Autodesk Fusion 360 part; units mm, degrees
note: some values were not read from the file. Set by a fixed rule: which sketch regions a step uses.
(part 2 of 2)
sketch "Sketch21" plane through (0, 0, -10) normal (0, 0, -1) x (1, 0, 0)
  spline S0 degree 3 poles (20.862, 26.2779) (22.0749, 27.628) (22.1899, 27.6698) (22.8451, 26.9999) knots 0 0 0 0 1 1 1 1
  spline S1 degree 3 poles (22.8451, 26.9999) (23.28, 26.5551) (23.2541, 26.3604) (22.6927, 25.8492) knots 0 0 0 0 1 1 1 1
  spline S2 degree 3 poles (22.6927, 25.8492) (21.2501, 24.5364) (20.8273, 24.3583) (20.2979, 24.842) knots 0 0 0 0 1 1 1 1
  spline S3 degree 3 poles (20.2979, 24.842) (19.869, 25.2336) (19.8267, 25.1253) (20.862, 26.2779) knots 0 0 0 0 1 1 1 1
  spline S4 degree 3 poles (14.6678, 20.2808) (15.0237, 20.7097) (15.5235, 21.3317) (17.1491, 23.3698) knots 0 0 0 0 1 1 1 1
  spline S5 degree 3 poles (17.1491, 23.3698) (17.5034, 23.8143) (17.8222, 24.1162) (17.9402, 24.1191) knots 0 0 0 0 1 1 1 1
  spline S6 degree 3 poles (17.9402, 24.1191) (18.2344, 24.1265) (19.9603, 22.9367) (20.9237, 22.0623) knots 0 0 0 0 1 1 1 1
  spline S7 degree 3 poles (20.9237, 22.0623) (20.9678, 22.0223) (20.8255, 21.7837) (20.6075, 21.5323) knots 0 0 0 0 1 1 1 1
  spline S8 degree 3 poles (20.6075, 21.5323) (20.3895, 21.2809) (19.9532, 20.7497) (19.6383, 20.3517) knots 0 0 0 0 1 1 1 1
  spline S9 degree 3 poles (19.6383, 20.3517) (18.9242, 19.4495) (17.0861, 17.5096) (16.9451, 17.5096) knots 0 0 0 0 1 1 1 1
  spline S10 degree 3 poles (16.9451, 17.5096) (16.8874, 17.5096) (16.566, 17.7633) (16.231, 18.0737) knots 0 0 0 0 1 1 1 1
  spline S11 degree 3 poles (16.231, 18.0737) (15.8958, 18.3838) (15.32, 18.8531) (14.9509, 19.1161) knots 0 0 0 0 1 1 1 1
  spline S12 degree 3 poles (14.9509, 19.1161) (14.1651, 19.677) (14.1654, 19.6755) (14.6678, 20.2808) knots 0 0 0 0 1 1 1 1
  spline S13 degree 3 poles (29.4215, 8.4259) (29.9899, 8.5418) (30.8969, 8.731) (31.4369, 8.8463) knots 0 0 0 0 1 1 1 1
  spline S14 degree 3 poles (31.4369, 8.8463) (31.9769, 8.9617) (32.628, 9.0921) (32.8839, 9.1363) knots 0 0 0 0 1 1 1 1
  spline S15 degree 3 poles (32.8839, 9.1363) (33.4104, 9.2273) (34.532, 9.444) (36.3462, 9.8054) knots 0 0 0 0 1 1 1 1
  spline S16 degree 3 poles (36.3462, 9.8054) (38.5867, 10.2521) (38.883, 10.3047) (38.9201, 10.2637) knots 0 0 0 0 1 1 1 1
  spline S17 degree 3 poles (38.9201, 10.2637) (39.3336, 9.807) (39.7083, 7.5488) (39.3982, 7.3826) knots 0 0 0 0 1 1 1 1
  spline S18 degree 3 poles (39.3982, 7.3826) (39.0804, 7.2128) (37.4413, 6.8204) (35.0543, 6.3428) knots 0 0 0 0 1 1 1 1
  spline S19 degree 3 poles (35.0543, 6.3428) (33.9459, 6.1211) (32.1086, 5.7496) (30.9717, 5.5173) knots 0 0 0 0 1 1 1 1
  spline S20 degree 3 poles (30.9717, 5.5173) (26.6447, 4.6334) (23.86, 4.1852) (23.7544, 4.3558) knots 0 0 0 0 1 1 1 1
  spline S21 degree 3 poles (23.7544, 4.3558) (23.6788, 4.4786) (23.2549, 6.4365) (23.2356, 6.7529) knots 0 0 0 0 1 1 1 1
  spline S22 degree 3 poles (23.2356, 6.7529) (23.2218, 6.9792) (23.2901, 7.0215) (23.9439, 7.1921) knots 0 0 0 0 1 1 1 1
  spline S23 degree 3 poles (23.9439, 7.1921) (25.0588, 7.4832) (27.5544, 8.0452) (29.4215, 8.4259) knots 0 0 0 0 1 1 1 1
  spline S24 degree 3 poles (31.5403, -12.6172) (31.5403, -12.6934) (31.5618, -12.8178) (31.5882, -12.8934) knots 0 0 0 0 1 1 1 1
  spline S25 degree 3 poles (31.5882, -12.8934) (31.6147, -12.9691) (31.5742, -13.1728) (31.4985, -13.3461) knots 0 0 0 0 1 1 1 1
  spline S26 degree 3 poles (31.4985, -13.3461) (31.0239, -14.4338) (29.3639, -14.115) (29.3734, -12.9379) knots 0 0 0 0 1 1 1 1
  spline S27 degree 3 poles (29.3734, -12.9379) (29.3813, -11.9494) (30.5288, -11.4671) (31.2223, -12.1605) knots 0 0 0 0 1 1 1 1
  spline S28 degree 3 poles (31.2223, -12.1605) (31.3972, -12.3354) (31.5403, -12.541) (31.5403, -12.6172) knots 0 0 0 0 1 1 1 1
  line L0 (15.4452, -28.439) -> (15.3796, -27.5151)
  spline S29 degree 3 poles (15.3796, -27.5151) (15.2729, -26.0133) (15.9352, -25.8345) (17.2002, -27.0232) knots 0 0 0 0 1 1 1 1
  spline S30 degree 3 poles (17.2002, -27.0232) (17.6648, -27.4601) (17.6664, -27.5019) (17.2568, -28.461) knots 0 0 0 0 1 1 1 1
  spline S31 degree 3 poles (17.2568, -28.461) (17.0798, -28.8756) (16.8843, -29.201) (16.8221, -29.1844) knots 0 0 0 0 1 1 1 1
  spline S32 degree 3 poles (16.8221, -29.1844) (16.7599, -29.1677) (16.4247, -28.9933) (16.077, -28.7965) knots 0 0 0 0 1 1 1 1
  line L1 (16.077, -28.7965) -> (15.4452, -28.439)
  line L2 (2.2258, -22.5912) -> (3.0868, -22.5912)
  line L3 (3.0868, -22.5912) -> (3.2683, -23.6506)
  spline S33 degree 3 poles (3.2683, -23.6506) (3.3683, -24.2332) (3.608, -25.3561) (3.8009, -26.1456) knots 0 0 0 0 1 1 1 1
  spline S34 degree 3 poles (3.8009, -26.1456) (4.2713, -28.0697) (4.2668, -28.1578) (3.6768, -28.6525) knots 0 0 0 0 1 1 1 1
  spline S35 degree 3 poles (3.6768, -28.6525) (3.0362, -29.1894) (2.588, -29.3391) (1.8387, -29.2659) knots 0 0 0 0 1 1 1 1
  spline S36 degree 3 poles (1.8387, -29.2659) (0.3557, -29.1206) (-0.1128, -28.1046) (0.4711, -26.2993) knots 0 0 0 0 1 1 1 1
  spline S37 degree 3 poles (0.4711, -26.2993) (0.6719, -25.6781) (1.0444, -24.1485) (1.3172, -22.8238) knots 0 0 0 0 1 1 1 1
  spline S38 degree 3 poles (1.3172, -22.8238) (1.3622, -22.6052) (1.4165, -22.5912) (2.2258, -22.5912) knots 0 0 0 0 1 1 1 1
  spline S39 degree 3 poles (-30.4455, 10.3042) (-30.1303, 10.7241) (-28.6807, 10.95) (-28.36, 10.6293) knots 0 0 0 0 1 1 1 1
  spline S40 degree 3 poles (-28.36, 10.6293) (-28.1904, 10.4597) (-28.0986, -8.8151) (-28.2666, -8.9832) knots 0 0 0 0 1 1 1 1
  spline S41 degree 3 poles (-28.2666, -8.9832) (-28.3537, -9.0702) (-29.8806, -9.0739) (-30.1049, -8.9879) knots 0 0 0 0 1 1 1 1
  spline S42 degree 3 poles (-30.1049, -8.9879) (-30.5796, -8.8056) (-30.5748, -8.9072) (-30.5748, 0.8967) knots 0 0 0 0 1 1 1 1
  spline S43 degree 3 poles (-30.5748, 0.8967) (-30.5748, 8.1243) (-30.5468, 10.1695) (-30.4455, 10.3042) knots 0 0 0 0 1 1 1 1
  spline S44 degree 3 poles (-13.179, 9.603) (-13.0383, 9.2054) (-12.7991, 8.4378) (-12.6472, 7.8978) knots 0 0 0 0 1 1 1 1
  spline S45 degree 3 poles (-12.6472, 7.8978) (-12.4951, 7.3578) (-12.349, 6.8389) (-12.3223, 6.7447) knots 0 0 0 0 1 1 1 1
  spline S46 degree 3 poles (-12.3223, 6.7447) (-12.104, 5.9769) (-17.0523, 3.5076) (-19.3094, 3.2581) knots 0 0 0 0 1 1 1 1
  line L4 (-19.3094, 3.2581) -> (-19.8777, 3.1953)
  line L5 (-19.8777, 3.1953) -> (-19.8777, -1.4539)
  line L6 (-19.8777, -1.4539) -> (-19.1025, -1.5682)
  spline S47 degree 3 poles (-19.1025, -1.5682) (-16.6231, -1.9341) (-13.6717, -3.4131) (-12.0702, -5.0925) knots 0 0 0 0 1 1 1 1
  spline S48 degree 3 poles (-12.0702, -5.0925) (-10.9073, -6.3114) (-9.4825, -8.0603) (-9.1812, -8.6387) knots 0 0 0 0 1 1 1 1
  spline S49 degree 3 poles (-9.1812, -8.6387) (-9.1071, -8.7808) (-9.0134, -8.9202) (-8.9729, -8.9488) knots 0 0 0 0 1 1 1 1
  spline S50 degree 3 poles (-8.9729, -8.9488) (-8.4647, -9.3062) (-8.1371, -13.3914) (-8.32, -17.0871) knots 0 0 0 0 1 1 1 1
  line L7 (-8.32, -17.0871) -> (-8.3623, -17.939)
  line L8 (-8.3623, -17.939) -> (-8.9568, -17.639)
  spline S51 degree 3 poles (-8.9568, -17.639) (-10.9986, -16.6085) (-12.788, -15.0109) (-14.5231, -12.6693) knots 0 0 0 0 1 1 1 1
  spline S52 degree 3 poles (-14.5231, -12.6693) (-16.5808, -9.8931) (-18.1228, -8.994) (-21.0377, -8.872) knots 0 0 0 0 1 1 1 1
  line L9 (-21.0377, -8.872) -> (-22.4098, -8.8144)
  line L10 (-22.4098, -8.8144) -> (-22.4098, 0.7612)
  spline S53 degree 3 poles (-22.4098, 0.7612) (-22.4098, 8.0711) (-22.3804, 10.3664) (-22.286, 10.4611) knots 0 0 0 0 1 1 1 1
  spline S54 degree 3 poles (-22.286, 10.4611) (-22.2063, 10.5404) (-21.8005, 10.5849) (-21.1557, 10.5849) knots 0 0 0 0 1 1 1 1
  spline S55 degree 3 poles (-21.1557, 10.5849) (-18.3574, 10.5849) (-15.9831, 11.8954) (-14.8821, 14.0472) knots 0 0 0 0 1 1 1 1
  spline S56 degree 3 poles (-14.8821, 14.0472) (-14.6784, 14.4457) (-14.5633, 14.5896) (-14.5602, 14.4494) knots 0 0 0 0 1 1 1 1
  spline S57 degree 3 poles (-14.5602, 14.4494) (-14.5541, 14.1856) (-13.5365, 10.6153) (-13.179, 9.603) knots 0 0 0 0 1 1 1 1
  spline S58 degree 3 poles (-5.6836, 12.591) (-5.958, 12.4497) (-5.9604, 12.4518) (-6.3298, 13.1654) knots 0 0 0 0 1 1 1 1
  spline S59 degree 3 poles (-6.3298, 13.1654) (-6.7885, 14.052) (-6.788, 14.0732) (-6.3128, 14.27) knots 0 0 0 0 1 1 1 1
  spline S60 degree 3 poles (-6.3128, 14.27) (-6.0996, 14.3584) (-5.7366, 14.5155) (-5.5061, 14.6198) knots 0 0 0 0 1 1 1 1
  spline S61 degree 3 poles (-5.5061, 14.6198) (-2.2832, 16.0763) (2.9227, 16.2012) (5.8226, 14.8915) knots 0 0 0 0 1 1 1 1
  spline S62 degree 3 poles (5.8226, 14.8915) (6.012, 14.8058) (6.4843, 14.5925) (6.8719, 14.4174) knots 0 0 0 0 1 1 1 1
  spline S63 degree 3 poles (6.8719, 14.4174) (7.2598, 14.2422) (7.5961, 14.0991) (7.6199, 14.0991) knots 0 0 0 0 1 1 1 1
  spline S64 degree 3 poles (7.6199, 14.0991) (8.0964, 14.0991) (10.6404, 12.052) (11.7939, 10.7399) knots 0 0 0 0 1 1 1 1
  spline S65 degree 3 poles (11.7939, 10.7399) (14.2884, 7.9039) (15.8315, 2.9054) (15.3518, -0.7837) knots 0 0 0 0 1 1 1 1
  spline S66 degree 3 poles (15.3518, -0.7837) (15.3261, -0.9827) (15.1899, -1.7124) (15.0494, -2.4054) knots 0 0 0 0 1 1 1 1
  spline S67 degree 3 poles (15.0494, -2.4054) (14.7007, -4.1254) (14.3112, -5.1134) (13.101, -7.348) knots 0 0 0 0 1 1 1 1
  spline S68 degree 3 poles (13.101, -7.348) (11.2545, -10.758) (6.6772, -13.6369) (2.5756, -13.9684) knots 0 0 0 0 1 1 1 1
  line L11 (2.5756, -13.9684) -> (1.6712, -14.0415)
  line L12 (1.6712, -14.0415) -> (1.6712, -13.6139)
  spline S69 degree 3 poles (1.6712, -13.6139) (1.6712, -13.3416) (1.7183, -13.1855) (1.8006, -13.1842) knots 0 0 0 0 1 1 1 1
  spline S70 degree 3 poles (1.8006, -13.1842) (8.8176, -13.0747) (14.7896, -6.5384) (14.4522, 0.663) knots 0 0 0 0 1 1 1 1
  spline S71 degree 3 poles (14.4522, 0.663) (13.9887, 10.5569) (3.0063, 17.0624) (-5.6836, 12.591) knots 0 0 0 0 1 1 1 1
  spline S72 degree 3 poles (-26.4402, 11.3101) (-26.1328, 12.3822) (-24.7717, 12.4981) (-24.26, 11.4953) knots 0 0 0 0 1 1 1 1
  spline S73 degree 3 poles (-24.26, 11.4953) (-24.0473, 11.0778) (-23.9563, -9.3226) (-24.1651, -9.8394) knots 0 0 0 0 1 1 1 1
  spline S74 degree 3 poles (-24.1651, -9.8394) (-24.5095, -10.6921) (-26.1336, -10.7379) (-26.4508, -9.9039) knots 0 0 0 0 1 1 1 1
  spline S75 degree 3 poles (-26.4508, -9.9039) (-26.5804, -9.5629) (-26.5704, 10.8564) (-26.4402, 11.3101) knots 0 0 0 0 1 1 1 1
  spline S76 degree 3 poles (4.9979, -22.0247) (5.0264, -21.9996) (7.2714, -21.4088) (7.8252, -21.2807) knots 0 0 0 0 1 1 1 1
  spline S77 degree 3 poles (7.8252, -21.2807) (8.0054, -21.2389) (8.0636, -21.3201) (8.2207, -21.834) knots 0 0 0 0 1 1 1 1
  spline S78 degree 3 poles (8.2207, -21.834) (9.0079, -24.4055) (11.1888, -31.0486) (12.3091, -34.2876) knots 0 0 0 0 1 1 1 1
  spline S79 degree 3 poles (12.3091, -34.2876) (12.5975, -35.1213) (12.8335, -35.8222) (12.8335, -35.8452) knots 0 0 0 0 1 1 1 1
  spline S80 degree 3 poles (12.8335, -35.8452) (12.8335, -35.8683) (12.6126, -35.9857) (12.3424, -36.1067) knots 0 0 0 0 1 1 1 1
  spline S81 degree 3 poles (12.3424, -36.1067) (10.7356, -36.8261) (10.1498, -37.0345) (10.0562, -36.9205) knots 0 0 0 0 1 1 1 1
  spline S82 degree 3 poles (10.0562, -36.9205) (10.003, -36.8554) (9.795, -36.3138) (9.5942, -35.7172) knots 0 0 0 0 1 1 1 1
  spline S83 degree 3 poles (9.5942, -35.7172) (9.3936, -35.1203) (8.9177, -33.7482) (8.5369, -32.6681) knots 0 0 0 0 1 1 1 1
  spline S84 degree 3 poles (8.5369, -32.6681) (7.8972, -30.8536) (6.5777, -27.0262) (5.8292, -24.8134) knots 0 0 0 0 1 1 1 1
  spline S85 degree 3 poles (5.8292, -24.8134) (5.4048, -23.5593) (4.9579, -22.0599) (4.9979, -22.0247) knots 0 0 0 0 1 1 1 1
  spline S86 degree 3 poles (21.0387, -22.9492) (21.6407, -22.859) (21.9426, -23.028) (22.962, -24.026) knots 0 0 0 0 1 1 1 1
  spline S87 degree 3 poles (22.962, -24.026) (23.964, -25.0066) (23.9616, -24.9203) (22.9998, -25.4686) knots 0 0 0 0 1 1 1 1
  spline S88 degree 3 poles (22.9998, -25.4686) (22.0664, -26.0006) (22.2111, -26.0856) (21.2099, -24.4197) knots 0 0 0 0 1 1 1 1
  spline S89 degree 3 poles (21.2099, -24.4197) (20.4003, -23.0722) (20.3971, -23.0455) (21.0387, -22.9492) knots 0 0 0 0 1 1 1 1
  line L13 (22.7035, -7.4025) -> (23.4271, -7.7206)
  spline S90 degree 3 poles (23.4271, -7.7206) (23.8251, -7.8957) (24.3831, -8.1471) (24.6672, -8.2794) knots 0 0 0 0 1 1 1 1
  spline S91 degree 3 poles (24.6672, -8.2794) (24.9517, -8.4114) (25.6025, -8.6911) (26.1142, -8.9003) knots 0 0 0 0 1 1 1 1
  spline S92 degree 3 poles (26.1142, -8.9003) (27.3837, -9.42) (28.1306, -9.7766) (28.1246, -9.8605) knots 0 0 0 0 1 1 1 1
  spline S93 degree 3 poles (28.1246, -9.8605) (28.1216, -9.8991) (27.9454, -10.3026) (27.7324, -10.7575) knots 0 0 0 0 1 1 1 1
  spline S94 degree 3 poles (27.7324, -10.7575) (27.5197, -11.212) (27.189, -11.9214) (26.9974, -12.3336) knots 0 0 0 0 1 1 1 1
  spline S95 degree 3 poles (26.9974, -12.3336) (26.5762, -13.2395) (26.5648, -13.2398) (24.9194, -12.3643) knots 0 0 0 0 1 1 1 1
  spline S96 degree 3 poles (24.9194, -12.3643) (24.8305, -12.3172) (24.0166, -11.9026) (23.1107, -11.443) knots 0 0 0 0 1 1 1 1
  spline S97 degree 3 poles (23.1107, -11.443) (22.2045, -10.9834) (21.4028, -10.5672) (21.3285, -10.5177) knots 0 0 0 0 1 1 1 1
  spline S98 degree 3 poles (21.3285, -10.5177) (21.2247, -10.4487) (21.3674, -10.0799) (21.9486, -8.9154) knots 0 0 0 0 1 1 1 1
  line L14 (21.9486, -8.9154) -> (22.7035, -7.4025)
  spline S99 degree 3 poles (33.5832, 1.5933) (34.3782, 1.5933) (34.8585, 0.8376) (34.5679, 0.0431) knots 0 0 0 0 1 1 1 1
  spline S100 degree 3 poles (34.5679, 0.0431) (34.242, -0.8485) (32.9074, -0.7922) (32.6291, 0.1249) knots 0 0 0 0 1 1 1 1
  spline S101 degree 3 poles (32.6291, 0.1249) (32.3986, 0.8837) (32.8598, 1.5933) (33.5832, 1.5933) knots 0 0 0 0 1 1 1 1
  spline S102 degree 3 poles (18.3254, 16.1044) (18.993, 16.6134) (22.1595, 18.9637) (22.4453, 19.1624) knots 0 0 0 0 1 1 1 1
  spline S103 degree 3 poles (22.4453, 19.1624) (22.6442, 19.3008) (22.8535, 19.4699) (22.9104, 19.5381) knots 0 0 0 0 1 1 1 1
  spline S104 degree 3 poles (22.9104, 19.5381) (22.9673, 19.6064) (23.1768, 19.771) (23.3763, 19.9038) knots 0 0 0 0 1 1 1 1
  spline S105 degree 3 poles (23.3763, 19.9038) (23.5756, 20.0366) (24.3116, 20.5637) (25.0117, 21.0754) knots 0 0 0 0 1 1 1 1
  spline S106 degree 3 poles (25.0117, 21.0754) (25.7116, 21.5868) (26.3857, 22.0739) (26.5093, 22.1575) knots 0 0 0 0 1 1 1 1
  spline S107 degree 3 poles (26.5093, 22.1575) (26.7807, 22.3406) (28.4087, 23.5318) (29.4562, 24.3136) knots 0 0 0 0 1 1 1 1
  line L15 (29.4562, 24.3136) -> (30.2142, 24.8793)
  line L16 (30.2142, 24.8793) -> (30.7418, 24.7573)
  spline S108 degree 3 poles (30.7418, 24.7573) (32.1319, 24.4366) (32.8736, 22.9925) (32.0311, 22.2477) knots 0 0 0 0 1 1 1 1
  spline S109 degree 3 poles (32.0311, 22.2477) (31.8464, 22.0845) (30.7979, 21.2886) (29.7007, 20.4795) knots 0 0 0 0 1 1 1 1
  spline S110 degree 3 poles (29.7007, 20.4795) (28.6037, 19.6704) (27.5517, 18.892) (27.3631, 18.7499) knots 0 0 0 0 1 1 1 1
  spline S111 degree 3 poles (27.3631, 18.7499) (27.1744, 18.6079) (26.5143, 18.1231) (25.896, 17.6728) knots 0 0 0 0 1 1 1 1
  spline S112 degree 3 poles (25.896, 17.6728) (25.2779, 17.2225) (24.7088, 16.7907) (24.6313, 16.7132) knots 0 0 0 0 1 1 1 1
  spline S113 degree 3 poles (24.6313, 16.7132) (24.5537, 16.6357) (24.2278, 16.3896) (23.9071, 16.1665) knots 0 0 0 0 1 1 1 1
  spline S114 degree 3 poles (23.9071, 16.1665) (23.5862, 15.9432) (22.626, 15.2469) (21.7735, 14.619) knots 0 0 0 0 1 1 1 1
  line L17 (21.7735, 14.619) -> (20.223, 13.4776)
  line L18 (20.223, 13.4776) -> (19.9648, 13.8014)
  spline S115 degree 3 poles (19.9648, 13.8014) (19.8227, 13.9798) (19.3623, 14.5454) (18.9417, 15.0582) knots 0 0 0 0 1 1 1 1
  spline S116 degree 3 poles (18.9417, 15.0582) (18.3106, 15.8279) (18.2027, 16.011) (18.3254, 16.1044) knots 0 0 0 0 1 1 1 1
  spline S117 degree 3 poles (5.041, 26.8875) (5.458, 28.5226) (5.9133, 30.2789) (6.053, 30.7906) knots 0 0 0 0 1 1 1 1
  spline S118 degree 3 poles (6.053, 30.7906) (6.1927, 31.302) (6.5406, 32.581) (6.8261, 33.6328) knots 0 0 0 0 1 1 1 1
  spline S119 degree 3 poles (6.8261, 33.6328) (8.0051, 37.9764) (8.1922, 38.4902) (8.5946, 38.4902) knots 0 0 0 0 1 1 1 1
  spline S120 degree 3 poles (8.5946, 38.4902) (9.0468, 38.4902) (10.9827, 37.6023) (10.9608, 37.4052) knots 0 0 0 0 1 1 1 1
  spline S121 degree 3 poles (10.9608, 37.4052) (10.9544, 37.3483) (10.5615, 35.7902) (10.0874, 33.9428) knots 0 0 0 0 1 1 1 1
  spline S122 degree 3 poles (10.0874, 33.9428) (9.6132, 32.0953) (9.1568, 30.2815) (9.0735, 29.9119) knots 0 0 0 0 1 1 1 1
  spline S123 degree 3 poles (9.0735, 29.9119) (8.6557, 28.0617) (7.3971, 23.2301) (7.3024, 23.1121) knots 0 0 0 0 1 1 1 1
  spline S124 degree 3 poles (7.3024, 23.1121) (7.2891, 23.0957) (7.0978, 23.1521) (6.8777, 23.2381) knots 0 0 0 0 1 1 1 1
  spline S125 degree 3 poles (6.8777, 23.2381) (6.5322, 23.3725) (5.4476, 23.6606) (4.5534, 23.8556) knots 0 0 0 0 1 1 1 1
  line L19 (4.5534, 23.8556) -> (4.2835, 23.9143)
  line L20 (4.2835, 23.9143) -> (5.041, 26.8875)
  line L21 (-0.2801, 34.5887) -> (-0.2925, 35.2864)
  line L22 (-0.2925, 35.2864) -> (0.1986, 35.307)
  spline S126 degree 3 poles (0.1986, 35.307) (1.0609, 35.3433) (1.2971, 35.3073) (1.435, 35.1186) knots 0 0 0 0 1 1 1 1
  spline S127 degree 3 poles (1.435, 35.1186) (1.6403, 34.8379) (1.7829, 34.2323) (1.6744, 34.1016) knots 0 0 0 0 1 1 1 1
  spline S128 degree 3 poles (1.6744, 34.1016) (1.6228, 34.0394) (1.5847, 33.8365) (1.59, 33.6507) knots 0 0 0 0 1 1 1 1
  spline S129 degree 3 poles (1.59, 33.6507) (1.6011, 33.2592) (1.5125, 33.1467) (1.1545, 33.0988) knots 0 0 0 0 1 1 1 1
  spline S130 degree 3 poles (1.1545, 33.0988) (0.8693, 33.0607) (0.8479, 32.8271) (0.9987, 31.3946) knots 0 0 0 0 1 1 1 1
  line L23 (0.9987, 31.3946) -> (1.0656, 30.7583)
  line L24 (1.0656, 30.7583) -> (1.7043, 30.6459)
  spline S131 degree 3 poles (1.7043, 30.6459) (2.6597, 30.4779) (3.0116, 30.1262) (2.8526, 29.4986) knots 0 0 0 0 1 1 1 1
  spline S132 degree 3 poles (2.8526, 29.4986) (2.8312, 29.4132) (2.7685, 28.5993) (2.7137, 27.6899) knots 0 0 0 0 1 1 1 1
  spline S133 degree 3 poles (2.7137, 27.6899) (2.6126, 26.0162) (2.4377, 24.6144) (2.2949, 24.3311) knots 0 0 0 0 1 1 1 1
  spline S134 degree 3 poles (2.2949, 24.3311) (2.2237, 24.1898) (-0.4422, 24.149) (-0.5901, 24.2869) knots 0 0 0 0 1 1 1 1
  spline S135 degree 3 poles (-0.5901, 24.2869) (-0.6722, 24.3633) (-1.1159, 28.5496) (-1.1175, 29.2616) knots 0 0 0 0 1 1 1 1
  line L25 (-1.1175, 29.2616) -> (-1.1193, 30.0066)
  line L26 (-1.1193, 30.0066) -> (-0.6648, 30.2728)
  spline S136 degree 3 poles (-0.6648, 30.2728) (-0.415, 30.4194) (-0.0078, 30.5736) (0.2396, 30.6154) knots 0 0 0 0 1 1 1 1
  spline S137 degree 3 poles (0.2396, 30.6154) (0.7621, 30.7043) (0.823, 30.9493) (0.6671, 32.3408) knots 0 0 0 0 1 1 1 1
  spline S138 degree 3 poles (0.6671, 32.3408) (0.5875, 33.052) (0.5798, 33.0663) (0.2242, 33.1808) knots 0 0 0 0 1 1 1 1
  spline S139 degree 3 poles (0.2242, 33.1808) (-0.1941, 33.3158) (-0.2613, 33.5034) (-0.2801, 34.5887) knots 0 0 0 0 1 1 1 1
  spline S140 degree 3 poles (9.6302, 23.2471) (9.9683, 23.9704) (10.2721, 24.7504) (10.8367, 26.3464) knots 0 0 0 0 1 1 1 1
  spline S141 degree 3 poles (10.8367, 26.3464) (11.301, 27.6582) (11.1788, 27.5934) (12.3189, 27.1346) knots 0 0 0 0 1 1 1 1
  spline S142 degree 3 poles (12.3189, 27.1346) (14.8602, 26.112) (14.988, 25.9866) (14.5416, 24.951) knots 0 0 0 0 1 1 1 1
  spline S143 degree 3 poles (14.5416, 24.951) (13.8572, 23.3632) (12.8158, 21.2952) (12.4723, 20.8415) knots 0 0 0 0 1 1 1 1
  spline S144 degree 3 poles (12.4723, 20.8415) (12.4308, 20.7864) (11.7246, 21.1254) (10.824, 21.6326) knots 0 0 0 0 1 1 1 1
  spline S145 degree 3 poles (10.824, 21.6326) (10.3154, 21.9186) (9.7691, 22.1816) (9.6095, 22.2165) knots 0 0 0 0 1 1 1 1
  spline S146 degree 3 poles (9.6095, 22.2165) (9.2436, 22.2969) (9.2463, 22.4261) (9.6302, 23.2471) knots 0 0 0 0 1 1 1 1
  spline S147 degree 3 poles (22.3442, 9.3869) (22.3423, 9.4578) (21.4819, 11.2911) (21.2385, 11.7422) knots 0 0 0 0 1 1 1 1
  spline S148 degree 3 poles (21.2385, 11.7422) (21.1896, 11.8332) (26.3783, 14.4092) (26.6101, 14.4092) knots 0 0 0 0 1 1 1 1
  spline S149 degree 3 poles (26.6101, 14.4092) (26.8159, 14.4092) (27.0001, 14.1345) (27.3033, 13.3755) knots 0 0 0 0 1 1 1 1
  spline S150 degree 3 poles (27.3033, 13.3755) (27.4282, 13.063) (27.6885, 12.4428) (27.8817, 11.9975) knots 0 0 0 0 1 1 1 1
  spline S151 degree 3 poles (27.8817, 11.9975) (28.2976, 11.0384) (28.2997, 11.0212) (28.0005, 10.8987) knots 0 0 0 0 1 1 1 1
  spline S152 degree 3 poles (28.0005, 10.8987) (27.8727, 10.8463) (27.326, 10.6336) (26.786, 10.4259) knots 0 0 0 0 1 1 1 1
  spline S153 degree 3 poles (26.786, 10.4259) (26.246, 10.2184) (25.7576, 10.0137) (25.701, 9.9708) knots 0 0 0 0 1 1 1 1
  spline S154 degree 3 poles (25.701, 9.9708) (25.601, 9.8959) (24.2693, 9.3591) (23.2348, 8.9768) knots 0 0 0 0 1 1 1 1
  line L27 (23.2348, 8.9768) -> (22.7323, 8.791)
  line L28 (22.7323, 8.791) -> (22.5395, 9.0421)
  spline S155 degree 3 poles (22.5395, 9.0421) (22.4334, 9.1802) (22.3455, 9.3353) (22.3442, 9.3869) knots 0 0 0 0 1 1 1 1
  spline S156 degree 3 poles (23.1811, -5.6857) (23.1184, -5.6161) (23.7126, -3.1007) (23.8452, -2.875) knots 0 0 0 0 1 1 1 1
  spline S157 degree 3 poles (23.8452, -2.875) (23.8542, -2.8596) (24.4847, -2.9898) (25.2462, -3.1642) knots 0 0 0 0 1 1 1 1
  spline S158 degree 3 poles (25.2462, -3.1642) (26.0079, -3.3385) (26.9686, -3.5481) (27.3813, -3.6296) knots 0 0 0 0 1 1 1 1
  spline S159 degree 3 poles (27.3813, -3.6296) (27.7941, -3.7113) (28.5847, -3.8902) (29.1384, -4.0272) knots 0 0 0 0 1 1 1 1
  spline S160 degree 3 poles (29.1384, -4.0272) (29.6919, -4.1643) (30.7961, -4.4257) (31.5919, -4.6083) knots 0 0 0 0 1 1 1 1
  spline S161 degree 3 poles (31.5919, -4.6083) (36.0499, -5.6306) (39.4024, -6.5403) (39.3844, -6.7226) knots 0 0 0 0 1 1 1 1
  spline S162 degree 3 poles (39.3844, -6.7226) (39.3786, -6.7816) (39.3085, -7.3184) (39.2286, -7.915) knots 0 0 0 0 1 1 1 1
  spline S163 degree 3 poles (39.2286, -7.915) (39.1487, -8.5119) (39.0619, -9.0586) (39.0357, -9.1295) knots 0 0 0 0 1 1 1 1
  spline S164 degree 3 poles (39.0357, -9.1295) (38.978, -9.2864) (37.93, -9.3046) (37.2963, -9.1596) knots 0 0 0 0 1 1 1 1
  spline S165 degree 3 poles (37.2963, -9.1596) (37.0579, -9.1051) (36.3745, -8.9477) (35.7776, -8.8096) knots 0 0 0 0 1 1 1 1
  spline S166 degree 3 poles (35.7776, -8.8096) (35.181, -8.6715) (34.2274, -8.4558) (33.6591, -8.3304) knots 0 0 0 0 1 1 1 1
  spline S167 degree 3 poles (33.6591, -8.3304) (33.0905, -8.205) (32.0907, -7.9685) (31.4369, -7.805) knots 0 0 0 0 1 1 1 1
  spline S168 degree 3 poles (31.4369, -7.805) (30.7833, -7.6415) (29.1787, -7.2509) (27.8713, -6.9371) knots 0 0 0 0 1 1 1 1
  spline S169 degree 3 poles (27.8713, -6.9371) (24.6392, -6.1614) (23.284, -5.7997) (23.1811, -5.6857) knots 0 0 0 0 1 1 1 1
  spline S170 degree 3 poles (15.9201, -16.859) (16.4525, -16.3738) (16.9253, -15.9766) (16.9708, -15.9766) knots 0 0 0 0 1 1 1 1
  spline S171 degree 3 poles (16.9708, -15.9766) (17.0697, -15.9766) (18.8054, -17.8403) (19.5153, -18.7084) knots 0 0 0 0 1 1 1 1
  spline S172 degree 3 poles (19.5153, -18.7084) (19.791, -19.0455) (20.3072, -19.6369) (20.6625, -20.0221) knots 0 0 0 0 1 1 1 1
  spline S173 degree 3 poles (20.6625, -20.0221) (21.4324, -20.8574) (21.4258, -20.8053) (20.8146, -21.2069) knots 0 0 0 0 1 1 1 1
  spline S174 degree 3 poles (20.8146, -21.2069) (20.5461, -21.3834) (20.0939, -21.6813) (19.8098, -21.8689) knots 0 0 0 0 1 1 1 1
  spline S175 degree 3 poles (19.8098, -21.8689) (18.15, -22.964) (18.2635, -22.9495) (17.6217, -22.152) knots 0 0 0 0 1 1 1 1
  spline S176 degree 3 poles (17.6217, -22.152) (15.4846, -19.4964) (14.7414, -18.5881) (14.5752, -18.4272) knots 0 0 0 0 1 1 1 1
  spline S177 degree 3 poles (14.5752, -18.4272) (14.321, -18.1819) (14.3324, -18.1197) (14.6678, -17.9147) knots 0 0 0 0 1 1 1 1
  spline S178 degree 3 poles (14.6678, -17.9147) (14.8242, -17.8194) (15.3878, -17.3443) (15.9201, -16.859) knots 0 0 0 0 1 1 1 1
  line L29 (2.9116, -32.8078) -> (2.9116, -33.9344)
  line L30 (2.9116, -33.9344) -> (2.3322, -33.9826)
  spline S179 degree 3 poles (2.3322, -33.9826) (1.2553, -34.0717) (0.9447, -33.7318) (0.9495, -32.4686) knots 0 0 0 0 1 1 1 1
  spline S180 degree 3 poles (0.9495, -32.4686) (0.9524, -31.6672) (1.7615, -31.2439) (2.6465, -31.5804) knots 0 0 0 0 1 1 1 1
  spline S181 degree 3 poles (2.6465, -31.5804) (2.9087, -31.6802) (2.9116, -31.6937) (2.9116, -32.8078) knots 0 0 0 0 1 1 1 1
  line L31 (-34.6058, 8.7762) -> (-32.229, 8.7762)
  line L32 (-32.229, 8.7762) -> (-32.2285, -7.0618)
  line L33 (-32.2285, -7.0618) -> (-32.7712, -7.1459)
  spline S182 degree 3 poles (-32.7712, -7.1459) (-33.3273, -7.2321) (-33.6803, -7.2292) (-34.2698, -7.1335) knots 0 0 0 0 1 1 1 1
  line L34 (-34.2698, -7.1335) -> (-34.6055, -7.0789)
  line L35 (-34.6055, -7.0789) -> (-34.6055, 0.8488)
  line L36 (-34.6055, 0.8488) -> (-34.6058, 8.7762)
  spline S183 degree 3 poles (-12.2763, 17.8713) (-12.5821, 18.5446) (-13.4457, 20.7714) (-14.6009, 23.8659) knots 0 0 0 0 1 1 1 1
  spline S184 degree 3 poles (-14.6009, 23.8659) (-14.7919, 24.3774) (-15.0986, 25.1912) (-15.2825, 25.6746) knots 0 0 0 0 1 1 1 1
  spline S185 degree 3 poles (-15.2825, 25.6746) (-15.4661, 26.1577) (-15.7923, 27.0415) (-16.0072, 27.6383) knots 0 0 0 0 1 1 1 1
  spline S186 degree 3 poles (-16.0072, 27.6383) (-16.222, 28.235) (-16.5906, 29.2351) (-16.8263, 29.8603) knots 0 0 0 0 1 1 1 1
  spline S187 degree 3 poles (-16.8263, 29.8603) (-17.062, 30.4855) (-17.3864, 31.3692) (-17.5473, 31.8241) knots 0 0 0 0 1 1 1 1
  spline S188 degree 3 poles (-17.5473, 31.8241) (-17.7082, 32.2789) (-17.9802, 33.0112) (-18.1519, 33.4518) knots 0 0 0 0 1 1 1 1
  spline S189 degree 3 poles (-18.1519, 33.4518) (-18.3238, 33.8923) (-18.4479, 34.2529) (-18.4278, 34.2529) knots 0 0 0 0 1 1 1 1
  spline S190 degree 3 poles (-18.4278, 34.2529) (-18.3731, 34.2529) (-16.9893, 31.3925) (-15.9278, 29.0851) knots 0 0 0 0 1 1 1 1
  spline S191 degree 3 poles (-15.9278, 29.0851) (-15.4661, 28.0821) (-15.1044, 27.3251) (-13.8534, 24.7443) knots 0 0 0 0 1 1 1 1
  spline S192 degree 3 poles (-13.8534, 24.7443) (-11.4023, 19.6876) (-11.3248, 19.5249) (-10.3662, 17.4064) knots 0 0 0 0 1 1 1 1
  spline S193 degree 3 poles (-10.3662, 17.4064) (-10.0961, 16.8095) (-9.8379, 16.2732) (-9.7924, 16.2144) knots 0 0 0 0 1 1 1 1
  spline S194 degree 3 poles (-9.7924, 16.2144) (-9.587, 15.9499) (-7.3783, 11.4117) (-6.7758, 10.0166) knots 0 0 0 0 1 1 1 1
  spline S195 degree 3 poles (-6.7758, 10.0166) (-6.4075, 9.1638) (-5.9347, 8.0708) (-5.7249, 7.5877) knots 0 0 0 0 1 1 1 1
  spline S196 degree 3 poles (-5.7249, 7.5877) (-4.801, 5.4589) (-3.1304, 0.9744) (-2.5571, -0.9152) knots 0 0 0 0 1 1 1 1
  spline S197 degree 3 poles (-2.5571, -0.9152) (-0.2491, -8.5244) (0.6209, -14.831) (0.0769, -20.0076) knots 0 0 0 0 1 1 1 1
  spline S198 degree 3 poles (0.0769, -20.0076) (-0.3444, -24.0133) (-1.1283, -26.7714) (-2.9489, -30.6528) knots 0 0 0 0 1 1 1 1
  spline S199 degree 3 poles (-2.9489, -30.6528) (-4.3184, -33.5727) (-6.3083, -37.6259) (-6.4398, -37.7635) knots 0 0 0 0 1 1 1 1
  spline S200 degree 3 poles (-6.4398, -37.7635) (-6.5991, -37.9302) (-9.0775, -36.8303) (-9.0775, -36.5932) knots 0 0 0 0 1 1 1 1
  spline S201 degree 3 poles (-9.0775, -36.5932) (-9.0775, -36.2477) (-7.7641, -33.3838) (-7.2291, -32.5631) knots 0 0 0 0 1 1 1 1
  spline S202 degree 3 poles (-7.2291, -32.5631) (-6.7793, -31.8725) (-6.7036, -31.7466) (-6.6084, -31.5291) knots 0 0 0 0 1 1 1 1
  spline S203 degree 3 poles (-6.6084, -31.5291) (-6.5578, -31.4143) (-6.2636, -30.8795) (-5.9543, -30.3406) knots 0 0 0 0 1 1 1 1
  spline S204 degree 3 poles (-5.9543, -30.3406) (-3.0111, -25.2146) (-1.6239, -17.399) (-2.5679, -11.2633) knots 0 0 0 0 1 1 1 1
  spline S205 degree 3 poles (-2.5679, -11.2633) (-3.1823, -7.2705) (-3.2881, -6.7514) (-4.1652, -3.4192) knots 0 0 0 0 1 1 1 1
  spline S206 degree 3 poles (-4.1652, -3.4192) (-4.9328, -0.5033) (-5.1645, 0.2675) (-5.7657, 1.9034) knots 0 0 0 0 1 1 1 1
  spline S207 degree 3 poles (-5.7657, 1.9034) (-6.0059, 2.5572) (-6.3882, 3.6036) (-6.6155, 4.2288) knots 0 0 0 0 1 1 1 1
  spline S208 degree 3 poles (-6.6155, 4.2288) (-6.8425, 4.854) (-7.3267, 6.0706) (-7.691, 6.9318) knots 0 0 0 0 1 1 1 1
  spline S209 degree 3 poles (-7.691, 6.9318) (-8.0556, 7.7933) (-8.3538, 8.5246) (-8.3538, 8.5571) knots 0 0 0 0 1 1 1 1
  spline S210 degree 3 poles (-8.3538, 8.5571) (-8.3538, 8.6122) (-9.3912, 11.0635) (-9.8024, 11.9803) knots 0 0 0 0 1 1 1 1
  spline S211 degree 3 poles (-9.8024, 11.9803) (-10.2033, 12.8735) (-11.2407, 15.3384) (-11.6077, 16.2695) knots 0 0 0 0 1 1 1 1
  spline S212 degree 3 poles (-11.6077, 16.2695) (-11.8207, 16.8095) (-12.1215, 17.5302) (-12.2763, 17.8713) knots 0 0 0 0 1 1 1 1
  spline S213 degree 3 poles (-8.3718, 16.6828) (-8.556, 17.0524) (-8.9777, 17.8607) (-9.309, 18.4793) knots 0 0 0 0 1 1 1 1
  spline S214 degree 3 poles (-9.309, 18.4793) (-9.6405, 19.0979) (-9.8966, 19.6188) (-9.8781, 19.6374) knots 0 0 0 0 1 1 1 1
  spline S215 degree 3 poles (-9.8781, 19.6374) (-9.8596, 19.6556) (-9.3116, 19.9085) (-8.6599, 20.1993) knots 0 0 0 0 1 1 1 1
  spline S216 degree 3 poles (-8.6599, 20.1993) (-2.9907, 22.729) (3.0204, 23.0952) (7.6455, 21.1928) knots 0 0 0 0 1 1 1 1
  spline S217 degree 3 poles (7.6455, 21.1928) (7.9694, 21.0598) (8.6793, 20.7806) (9.223, 20.5729) knots 0 0 0 0 1 1 1 1
  spline S218 degree 3 poles (9.223, 20.5729) (11.1619, 19.8326) (13.6317, 18.1652) (15.6751, 16.2176) knots 0 0 0 0 1 1 1 1
  spline S219 degree 3 poles (15.6751, 16.2176) (15.922, 15.9827) (17.2713, 14.4301) (17.7526, 13.8276) knots 0 0 0 0 1 1 1 1
  spline S220 degree 3 poles (17.7526, 13.8276) (19.0184, 12.2433) (20.3514, 9.8076) (20.9977, 7.8978) knots 0 0 0 0 1 1 1 1
  spline S221 degree 3 poles (20.9977, 7.8978) (21.1803, 7.3578) (21.3671, 6.8231) (21.4126, 6.7093) knots 0 0 0 0 1 1 1 1
  spline S222 degree 3 poles (21.4126, 6.7093) (21.5449, 6.3783) (21.919, 4.6241) (22.0849, 3.557) knots 0 0 0 0 1 1 1 1
  spline S223 degree 3 poles (22.0849, 3.557) (22.3, 2.1751) (22.2741, -0.8229) (22.0352, -2.2307) knots 0 0 0 0 1 1 1 1
  spline S224 degree 3 poles (22.0352, -2.2307) (20.7948, -9.5377) (16.5451, -15.4128) (10.3012, -18.4521) knots 0 0 0 0 1 1 1 1
  spline S225 degree 3 poles (10.3012, -18.4521) (8.1054, -19.521) (4.7206, -20.4399) (2.4052, -20.5955) knots 0 0 0 0 1 1 1 1
  line L37 (2.4052, -20.5955) -> (1.4339, -20.6608)
  line L38 (1.4339, -20.6608) -> (1.4942, -20.4116)
  spline S226 degree 3 poles (1.4942, -20.4116) (1.6437, -19.7967) (1.7959, -17.4908) (1.7445, -16.6227) knots 0 0 0 0 1 1 1 1
  line L39 (1.7445, -16.6227) -> (1.6879, -15.6665)
  line L40 (1.6879, -15.6665) -> (2.0991, -15.6665)
  spline S227 degree 3 poles (2.0991, -15.6665) (3.5506, -15.6665) (6.3806, -14.8667) (8.2779, -13.9198) knots 0 0 0 0 1 1 1 1
  spline S228 degree 3 poles (8.2779, -13.9198) (11.9368, -12.0941) (14.8665, -8.776) (16.3178, -4.8146) knots 0 0 0 0 1 1 1 1
  spline S229 degree 3 poles (16.3178, -4.8146) (18.4887, 1.1118) (17.0068, 7.8131) (12.485, 12.5182) knots 0 0 0 0 1 1 1 1
  spline S230 degree 3 poles (12.485, 12.5182) (7.8159, 17.3767) (0.6846, 18.8441) (-5.8733, 16.2959) knots 0 0 0 0 1 1 1 1
  spline S231 degree 3 poles (-5.8733, 16.2959) (-7.9556, 15.4871) (-7.7614, 15.4569) (-8.3718, 16.6828) knots 0 0 0 0 1 1 1 1
  spline S232 degree 3 poles (-11.0753, 6.1925) (-11.3203, 7.1316) (-11.994, 9.4215) (-12.5268, 11.1268) knots 0 0 0 0 1 1 1 1
  spline S233 degree 3 poles (-12.5268, 11.1268) (-13.1825, 13.226) (-13.8794, 16.5663) (-13.6989, 16.7465) knots 0 0 0 0 1 1 1 1
  spline S234 degree 3 poles (-13.6989, 16.7465) (-13.6759, 16.7698) (-13.5492, 16.3811) (-13.4177, 15.8832) knots 0 0 0 0 1 1 1 1
  spline S235 degree 3 poles (-13.4177, 15.8832) (-13.1597, 14.9066) (-13.1674, 14.9275) (-12.0884, 12.2385) knots 0 0 0 0 1 1 1 1
  spline S236 degree 3 poles (-12.0884, 12.2385) (-11.356, 10.414) (-10.3107, 7.7951) (-9.3656, 5.4173) knots 0 0 0 0 1 1 1 1
  spline S237 degree 3 poles (-9.3656, 5.4173) (-9.083, 4.7069) (-8.6668, 3.6139) (-8.4406, 2.9884) knots 0 0 0 0 1 1 1 1
  spline S238 degree 3 poles (-8.4406, 2.9884) (-8.2144, 2.3632) (-7.9437, 1.6192) (-7.8395, 1.3348) knots 0 0 0 0 1 1 1 1
  spline S239 degree 3 poles (-7.8395, 1.3348) (-7.7352, 1.0506) (-7.5744, 0.6088) (-7.4823, 0.3532) knots 0 0 0 0 1 1 1 1
  spline S240 degree 3 poles (-7.4823, 0.3532) (-7.3902, 0.0973) (-7.273, -0.2051) (-7.2217, -0.3188) knots 0 0 0 0 1 1 1 1
  spline S241 degree 3 poles (-7.2217, -0.3188) (-7.0436, -0.7144) (-6.2578, -3.2877) (-5.7228, -5.2279) knots 0 0 0 0 1 1 1 1
  spline S242 degree 3 poles (-5.7228, -5.2279) (-5.2958, -6.776) (-4.6314, -10.4921) (-4.4848, -12.1526) knots 0 0 0 0 1 1 1 1
  spline S243 degree 3 poles (-4.4848, -12.1526) (-4.4121, -12.976) (-4.3303, -17.5231) (-4.3819, -17.8888) knots 0 0 0 0 1 1 1 1
  spline S244 degree 3 poles (-4.3819, -17.8888) (-4.4057, -18.0592) (-4.475, -18.7103) (-4.5356, -19.3358) knots 0 0 0 0 1 1 1 1
  spline S245 degree 3 poles (-4.5356, -19.3358) (-5.4212, -28.4747) (-10.7163, -33.8318) (-14.8388, -29.7585) knots 0 0 0 0 1 1 1 1
  spline S246 degree 3 poles (-14.8388, -29.7585) (-17.0472, -27.5765) (-19.0536, -22.2867) (-19.8243, -16.6137) knots 0 0 0 0 1 1 1 1
  spline S247 degree 3 poles (-19.8243, -16.6137) (-20.1786, -14.0055) (-20.4445, -11.7859) (-20.4138, -11.6935) knots 0 0 0 0 1 1 1 1
  spline S248 degree 3 poles (-20.4138, -11.6935) (-20.3937, -11.6338) (-20.3442, -11.7938) (-20.3035, -12.0494) knots 0 0 0 0 1 1 1 1
  spline S249 degree 3 poles (-20.3035, -12.0494) (-20.2627, -12.3053) (-19.9748, -13.5374) (-19.6637, -14.7881) knots 0 0 0 0 1 1 1 1
  spline S250 degree 3 poles (-19.6637, -14.7881) (-17.7653, -22.4184) (-16.2302, -25.4431) (-13.5545, -26.8256) knots 0 0 0 0 1 1 1 1
  spline S251 degree 3 poles (-13.5545, -26.8256) (-8.3676, -29.5056) (-4.969, -16.7855) (-7.936, -5.7965) knots 0 0 0 0 1 1 1 1
  spline S252 degree 3 poles (-7.936, -5.7965) (-8.0435, -5.3986) (-8.2329, -4.5614) (-8.3573, -3.936) knots 0 0 0 0 1 1 1 1
  spline S253 degree 3 poles (-8.3573, -3.936) (-8.57, -2.867) (-8.9176, -1.4648) (-9.3828, 0.1982) knots 0 0 0 0 1 1 1 1
  spline S254 degree 3 poles (-9.3828, 0.1982) (-9.4942, 0.5958) (-9.7442, 1.5028) (-9.9387, 2.2135) knots 0 0 0 0 1 1 1 1
  spline S255 degree 3 poles (-9.9387, 2.2135) (-10.1329, 2.9239) (-10.4319, 3.9703) (-10.6028, 4.5389) knots 0 0 0 0 1 1 1 1
  spline S256 degree 3 poles (-10.6028, 4.5389) (-10.7737, 5.1072) (-10.9864, 5.8515) (-11.0753, 6.1925) knots 0 0 0 0 1 1 1 1
  spline S257 degree 3 poles (-38.7396, 0.763) (-38.7396, 3.465) (-38.7026, 4.8802) (-38.628, 5.0194) knots 0 0 0 0 1 1 1 1
  spline S258 degree 3 poles (-38.628, 5.0194) (-38.3658, 5.5097) (-37.0569, 5.6004) (-36.5724, 5.162) knots 0 0 0 0 1 1 1 1
  spline S259 degree 3 poles (-36.5724, 5.162) (-36.2433, 4.8641) (-36.2441, -3.4351) (-36.5732, -3.7328) knots 0 0 0 0 1 1 1 1
  spline S260 degree 3 poles (-36.5732, -3.7328) (-36.9992, -4.1185) (-37.9506, -4.0741) (-38.3761, -3.6486) knots 0 0 0 0 1 1 1 1
  line L41 (-38.3761, -3.6486) -> (-38.7396, -3.2848)
  line L42 (-38.7396, -3.2848) -> (-38.7396, 0.763)
  spline S261 degree 3 poles (10.5083, -22.5367) (10.0818, -21.6501) (9.7328, -20.8841) (9.7328, -20.8346) knots 0 0 0 0 1 1 1 1
  spline S262 degree 3 poles (9.7328, -20.8346) (9.7328, -20.6978) (12.7554, -19.0601) (12.8377, -19.1522) knots 0 0 0 0 1 1 1 1
  spline S263 degree 3 poles (12.8377, -19.1522) (12.9274, -19.2524) (14.5165, -22.2896) (14.9888, -23.263) knots 0 0 0 0 1 1 1 1
  spline S264 degree 3 poles (14.9888, -23.263) (15.1817, -23.6609) (15.4269, -24.1099) (15.5336, -24.261) knots 0 0 0 0 1 1 1 1
  spline S265 degree 3 poles (15.5336, -24.261) (15.7849, -24.6166) (15.7802, -24.6428) (15.4431, -24.774) knots 0 0 0 0 1 1 1 1
  spline S266 degree 3 poles (15.4431, -24.774) (15.2867, -24.8346) (14.7806, -25.019) (14.3183, -25.1833) knots 0 0 0 0 1 1 1 1
  spline S267 degree 3 poles (14.3183, -25.1833) (13.8561, -25.3479) (13.1833, -25.6217) (12.8232, -25.7921) knots 0 0 0 0 1 1 1 1
  line L43 (12.8232, -25.7921) -> (12.1681, -26.102)
  line L44 (12.1681, -26.102) -> (11.9773, -25.7159)
  spline S268 degree 3 poles (11.9773, -25.7159) (11.8725, -25.5037) (11.6733, -25.0643) (11.5352, -24.7396) knots 0 0 0 0 1 1 1 1
  spline S269 degree 3 poles (11.5352, -24.7396) (11.3968, -24.4147) (10.9346, -23.4233) (10.5083, -22.5367) knots 0 0 0 0 1 1 1 1
  spline S270 degree 3 poles (20.5461, -12.282) (20.7096, -12.4145) (20.9829, -12.6103) (21.1533, -12.717) knots 0 0 0 0 1 1 1 1
  spline S271 degree 3 poles (21.1533, -12.717) (21.324, -12.8233) (22.1765, -13.4493) (23.0483, -14.1076) knots 0 0 0 0 1 1 1 1
  spline S272 degree 3 poles (23.0483, -14.1076) (23.9198, -14.7662) (24.858, -15.4676) (25.1329, -15.6665) knots 0 0 0 0 1 1 1 1
  spline S273 degree 3 poles (25.1329, -15.6665) (25.4075, -15.8655) (26.2704, -16.5166) (27.0501, -17.1135) knots 0 0 0 0 1 1 1 1
  spline S274 degree 3 poles (27.0501, -17.1135) (27.8298, -17.7104) (28.659, -18.3357) (28.8929, -18.5029) knots 0 0 0 0 1 1 1 1
  spline S275 degree 3 poles (28.8929, -18.5029) (32.5169, -21.0937) (32.7132, -21.3347) (32.1333, -22.4788) knots 0 0 0 0 1 1 1 1
  spline S276 degree 3 poles (32.1333, -22.4788) (31.8422, -23.0526) (31.2183, -23.5215) (30.7455, -23.5215) knots 0 0 0 0 1 1 1 1
  spline S277 degree 3 poles (30.7455, -23.5215) (30.1812, -23.5215) (29.825, -23.2918) (26.5082, -20.7902) knots 0 0 0 0 1 1 1 1
  spline S278 degree 3 poles (26.5082, -20.7902) (25.6094, -20.1121) (23.6647, -18.6508) (22.1868, -17.5427) knots 0 0 0 0 1 1 1 1
  spline S279 degree 3 poles (22.1868, -17.5427) (18.998, -15.1517) (18.3588, -14.6394) (18.3749, -14.4881) knots 0 0 0 0 1 1 1 1
  spline S280 degree 3 poles (18.3749, -14.4881) (18.3895, -14.3537) (20.0497, -12.1145) (20.1675, -12.0708) knots 0 0 0 0 1 1 1 1
  spline S281 degree 3 poles (20.1675, -12.0708) (20.2122, -12.0542) (20.3826, -12.1492) (20.5461, -12.282) knots 0 0 0 0 1 1 1 1
  line L45 (24.0989, 0.7683) -> (24.0989, 2.3167)
  line L46 (24.0989, 2.3167) -> (29.8867, 2.3167)
  line L47 (29.8867, 2.3167) -> (29.8692, 0.8956)
  spline S282 degree 3 poles (29.8692, 0.8956) (29.8597, 0.114) (29.8335, -0.7046) (29.8107, -0.9237) knots 0 0 0 0 1 1 1 1
  line L48 (29.8107, -0.9237) -> (29.7695, -1.3219)
  line L49 (29.7695, -1.3219) -> (28.717, -1.2534)
  spline S283 degree 3 poles (28.717, -1.2534) (27.403, -1.1682) (24.6424, -0.903) (24.3315, -0.8327) knots 0 0 0 0 1 1 1 1
  spline S284 degree 3 poles (24.3315, -0.8327) (24.1029, -0.7808) (24.0989, -0.7528) (24.0989, 0.7683) knots 0 0 0 0 1 1 1 1
  spline S285 degree 3 poles (30.4412, 15.4426) (31.2681, 15.4426) (31.7814, 14.6145) (31.4432, 13.8258) knots 0 0 0 0 1 1 1 1
  spline S286 degree 3 poles (31.4432, 13.8258) (31.2326, 13.3342) (30.2931, 13.0807) (29.8819, 13.4046) knots 0 0 0 0 1 1 1 1
  spline S287 degree 3 poles (29.8819, 13.4046) (28.9707, 14.1226) (29.3329, 15.4426) (30.4412, 15.4426) knots 0 0 0 0 1 1 1 1
  line L50 (13.4767, 28.603) -> (13.8236, 29.2941)
  spline S288 degree 3 poles (13.8236, 29.2941) (14.916, 31.4711) (16.7877, 31.0263) (15.791, 28.8269) knots 0 0 0 0 1 1 1 1
  spline S289 degree 3 poles (15.791, 28.8269) (15.2341, 27.5976) (15.3735, 27.6622) (14.3609, 28.1643) knots 0 0 0 0 1 1 1 1
  line L51 (14.3609, 28.1643) -> (13.4767, 28.603)
  spline S290 degree 3 poles (-7.3204, 37.8145) (-7.3204, 37.7298) (-7.2767, 37.5798) (-7.2235, 37.4811) knots 0 0 0 0 1 1 1 1
  spline S291 degree 3 poles (-7.2235, 37.4811) (-7.1703, 37.3824) (-6.7486, 36.2786) (-6.2861, 35.0279) knots 0 0 0 0 1 1 1 1
  spline S292 degree 3 poles (-6.2861, 35.0279) (-5.8239, 33.7775) (-5.1719, 32.0333) (-4.8372, 31.1523) knots 0 0 0 0 1 1 1 1
  spline S293 degree 3 poles (-4.8372, 31.1523) (-3.1161, 26.6194) (-2.2113, 23.9215) (-2.3954, 23.8699) knots 0 0 0 0 1 1 1 1
  spline S294 degree 3 poles (-2.3954, 23.8699) (-2.8272, 23.7492) (-5.2881, 23.1973) (-5.2981, 23.219) knots 0 0 0 0 1 1 1 1
  spline S295 degree 3 poles (-5.2981, 23.219) (-5.3048, 23.2336) (-5.6059, 24.1527) (-5.9673, 25.2611) knots 0 0 0 0 1 1 1 1
  spline S296 degree 3 poles (-5.9673, 25.2611) (-6.3284, 26.3697) (-7.042, 28.416) (-7.5527, 29.8087) knots 0 0 0 0 1 1 1 1
  spline S297 degree 3 poles (-7.5527, 29.8087) (-10.0091, 36.5072) (-10.1831, 37.0054) (-10.0977, 37.0911) knots 0 0 0 0 1 1 1 1
  spline S298 degree 3 poles (-10.0977, 37.0911) (-9.8098, 37.379) (-7.3204, 38.0275) (-7.3204, 37.8145) knots 0 0 0 0 1 1 1 1
  line L52 (-40, 40) -> (-40, -40)
  line L53 (-40, -40) -> (40, -40)
  line L54 (40, -40) -> (40, 40)
  line L55 (40, 40) -> (-40, 40)
  line L56 (30, 30) -> (-30, 30)
  line L57 (-30, 30) -> (-30, -30)
  line L58 (-30, -30) -> (30, -30)
  line L59 (30, -30) -> (30, 30)
  line L60 (30, 30) -> (-30, -30) construction
  line L61 (-30, 30) -> (30, -30) construction
  dimension "d160" = 60
  dimension "d161" = 60
  constraint horizontal L56
  constraint perpendicular L56 L57
  constraint parallel L56 L58
  constraint parallel L57 L59
  constraint coincident L60 origin
  constraint coincident L61 origin
  measures "d160" distance of L57.end L58.end
  measures "d161" distance of L56.end L57.end
hole "Hole7" at (30, 30, -10) at (-30, 30, -10) at (-30, -30, -10) at (30, -30, -10) direction (0, 0, 1) diameter 2.529 depth 4 tip angle 180 bodies 1
thread "Thread4" "ISO Metric profile 3.0 M3x0.5 6H"
sketch "Sketch22" plane through (-40, 0, 0) normal (1, 0, 0) x (0, 1, 0)
  line L0 (40, -10) -> (-40, -10)
  line L1 (-40, -10) -> (-40, -40)
  line L2 (-40, -40) -> (40, -40)
  line L3 (40, -40) -> (40, -10)
  line L4 (20, -33) -> (-8, -33)
  line L5 (-8, -33) -> (-8, -17)
  line L6 (-8, -17) -> (20, -17)
  line L7 (20, -17) -> (20, -33)
  line L8 (20, -33) -> (-8, -17) construction
  line L9 (-8, -33) -> (20, -17) construction
  circle A0 centre (0, -25) radius 6
  line L10 (40, -25) -> (-40, -25)
  point P0 (6, -25)
  dimension "d166" = 28
  dimension "d167" = 16
  dimension "d169" = 12
  dimension "d170" = 6
  constraint horizontal L4
  constraint perpendicular L4 L5
  constraint parallel L4 L6
  constraint parallel L5 L7
  constraint coincident L8 P0
  constraint coincident L9 P0
  constraint horizontal P0 A0.centre
  constraint coincident L3 L10.start
  constraint coincident L1 L10.end
  constraint midpoint L3 L10.start
  constraint midpoint L1 L10.end
  constraint midpoint A0.centre L10
  measures "d166" distance of L5.end L6.end
  measures "d167" distance of L4.start L6.end
  measures "d169" diameter of A0
  measures "d170" distance of P0 A0.centre
extrude "Extrude11" cut sketch "Sketch22" against normal blind 13 contours L5 L6 L7 A0 L10 | L4 L5 L7 A0 L10 bodies 1
extrude "Extrude12" cut sketch "Sketch22" against normal through all contours A0 L10 | A0 L10 bodies 1
